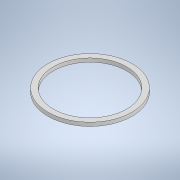
# Autodesk Inventor part: partDoc
Saved by Autodesk Inventor 2020 (Build 240168000, 168)
## iProperties
Created: 2020-06-26
Part Number: partDoc
Material: Generic
Document SubType Name: Modeling
Designer: minso
Density: 1 g/cm^3
Appearance: Default
Author: minso
Autodesk Inventor part; units mm, degrees
ref_plane "YZ Plane" through (0, 0, 0) normal (1, 0, 0) x (0, 1, 0)
ref_plane "XZ Plane" through (0, 0, 0) normal (0, 1, 0) x (-1, 0, 0)
ref_plane "XY Plane" through (0, 0, 0) normal (0, 0, 1) x (1, 0, 0)
sketch "Sketch2" plane through (0, 0, 0) normal (1, 0, 0) x (0, 1, 0)
  line L0 (5, 114.8) -> (-5, 114.8)
  line L1 (-5, 114.8) -> (-5, 100.2)
  line L2 (-5, 100.2) -> (5, 100.2)
  line L3 (5, 100.2) -> (5, 114.8)
  line L4 (13.1651, 0) -> (-13.1651, 0)
  point P0 (0, 0)
  point P1 (0, 0)
  point P2 (0, 100.2)
  dimension "height" = 10
  dimension "crossSection" = 14.6
  dimension "externalDiameter_coll" = 229.6
  constraints: 10 end point, 2 coincident, 2 horizontal, 2 midpoint, 2 parallel, 1 perpendicular, 1 vertical alignment
  measures "height" distance of L0.start L0.end
  measures "crossSection" distance between parallel lines of L2 L0
  measures "externalDiameter_coll" diameter of L0 L4
revolve "Revolution1" add sketch "Sketch2" angle 360 about axis through (0, 13.1651, 0) along (0, -1, 0)
body "Solid1"
